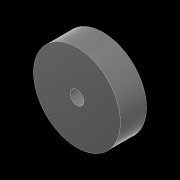
# Autodesk Inventor part: WheelMockup
Saved by Autodesk Inventor 2022 (Build 260153000, 153)
## iProperties
Created: 2022-10-07
Part Number: WheelMockup
Material: Generic
Document SubType Name: Modeling
Designer: tandu
Density: 0.108781 g/cm^3
Appearance: Smooth - Black
Mass: 6.4 g
Surface Area: 105.755 cm^2
Volume: 58.8337 cm^3
Author: tandu
Autodesk Inventor part; units mm, degrees
ref_plane "YZ Plane" through (0, 0, 0) normal (1, 0, 0) x (0, 1, 0)
ref_plane "XZ Plane" through (0, 0, 0) normal (0, 1, 0) x (-1, 0, 0)
ref_plane "XY Plane" through (0, 0, 0) normal (0, 0, 1) x (1, 0, 0)
sketch "Sketch1" plane through (0, 0, 0) normal (0, 0, 1) x (1, 0, 0)
  circle A0 centre (0, 0) radius 5
  circle A1 centre (0, 0) radius 31.75
  dimension "d0" = 10
  dimension "d1" = 63.5
  constraints: 2 centre point, 2 coincident
  measures "d0" diameter of A0
  measures "d1" diameter of A1
extrude "Extrusion1" add sketch "Sketch1" along normal blind 19.05
equation "\"d1\" = WheelDiameter"
equation "\"d2\" = WheelWidth"
equation "\"WheelDiameter\" = 63.5"
equation "\"WheelWidth\" = 19.05"
body "Solid1"
